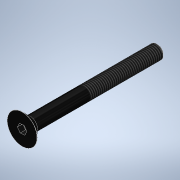
# Autodesk Inventor part: SCREW,FLAT HD,P, 5,M8X1.25X100MM
Saved by Autodesk Inventor 2022.4 (Build 264492000, 492)
## iProperties
Category: _
Manager: 608-09748
Created: 2001-02-21
Part Number: SCREW,FLAT HD,P, 5,M8X1.25X100MM
Material: Default
Document SubType Name: Modeling
Designer: cdotson
Description: SCREW,FLAT HD,P, 5,M8X1.25X100MM
Density: 1 g/cm^3
Appearance: Glossy - Black
Checked By: 0001244733
User Status: Released
Engr Approved By: P
Mfg Approved By: -
Mass: 8.56714 g
Surface Area: 39.1178 cm^2
Volume: 8.56714 cm^3
Control State: 0
Master: False
Checked Out: False
Shininess: 64.0
Length Units: 11269
Angle Units: 11279
Time Units: 11290
Mass Units: 11283
Length Display Precision: 3
Angle Display Precision: 2
PTC_WM_ITERATION: 1
PTC_WM_ORGANIZATION_ID: CLWC
PTC_WM_LIFECYCLE: CLWC_CAD_LC
FIRST_DESCRIPTION: _
SECOND_DESCRIPTION: _
THIRD_DESCRIPTION: _
CN_MASS: 0.008567
CL_runCount: 1
FinishProperty: ToBeSet
CN_Serviceable: _
Density: 0.0
Volumn: 0.0
Area: 0.0
PropertySet Name: Model Information
Subject: _
Author: -
Keywords: FASTENAL
Revision Number: A
Autodesk Inventor part; units mm, degrees
ref_plane "YZ Plane" through (0, 0, 0) normal (1, 0, 0) x (0, 1, 0)
ref_plane "XZ Plane" through (0, 0, 0) normal (0, 1, 0) x (-1, 0, 0)
ref_plane "XY Plane" through (0, 0, 0) normal (0, 0, 1) x (1, 0, 0)
sketch "Sketch1" plane through (0, 0, 0) normal (0, 0, 1) x (1, 0, 0)
  circle A0 centre (0, 0) radius 5
  dimension "Diameter" = 10
  constraints: 1 centre point
  measures "Diameter" diameter of A0
extrude "Extrusion1" add sketch "Sketch1" along normal blind 93.8
sketch "Sketch2" plane through (0, 0, 93.8) normal (0, 0, 1) x (1, 0, 0)
  circle A0 centre (0, 0) radius 5 projected
extrude "Extrusion2" add sketch "Sketch2" along normal blind 6.2 draft 45
sketch "Sketch3" plane through (0, 0, 100) normal (0, 0, 1) x (1, 0, 0)
  circle A0 centre (0, 0) radius 11.2 projected
  circle A1 centre (0, 0) radius 3.4641 construction
  line L0 (1.4501, 3.146) -> (3.4495, 0.3172)
  line L1 (3.4495, 0.3172) -> (1.9995, -2.8288)
  line L2 (1.9995, -2.8288) -> (-1.4501, -3.146)
  line L3 (-1.4501, -3.146) -> (-3.4495, -0.3172)
  line L4 (-3.4495, -0.3172) -> (-1.9995, 2.8288)
  line L5 (-1.9995, 2.8288) -> (1.4501, 3.146)
  dimension "Hex_Width" = 6
  constraints: 12 end point, 6 point on circle, 4 equal length, 1 centre point, 1 coincident
  measures "Hex_Width" distance between parallel lines of L0 L3
extrude "Extrusion3" cut sketch "Sketch3" against normal blind 4 contours L0 L1 L2 L3 L4 L5
thread "Thread1" size "M10x1.5" class "4g6g" standard "ANSI Metric M Profile" length 55
chamfer "Chamfer2" distance 1 angle 45 1 edges at (-5, 0, 0)
fillet "Fillet1" radius 0.1 1 edges at (-11.2, 0, 100)
equation "\"d10\" = Thread_Length"
equation "\"d13\" = Chamfer"
equation "\"Thread_Length\" = 55"
equation "\"Chamfer\" = 1"
body "Solid1"
